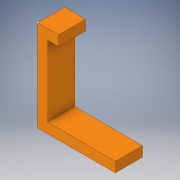
# Autodesk Inventor part: door stop supreme
Saved by Autodesk Inventor 2017 (Build 210142000, 142)
## iProperties
Created: 2018-09-26
Part Number: door stop supreme
Material: Generic
Document SubType Name: Modeling
Designer: Delta
Density: 1 g/cm^3
Appearance: Orange
Author: Delta
Autodesk Inventor part; units mm, degrees
ref_plane "YZ Plane" through (0, 0, 0) normal (1, 0, 0) x (0, 1, 0)
ref_plane "XZ Plane" through (0, 0, 0) normal (0, 1, 0) x (-1, 0, 0)
ref_plane "XY Plane" through (0, 0, 0) normal (0, 0, 1) x (1, 0, 0)
sketch "Sketch1" plane through (0, 0, 0) normal (0, 0, 1) x (1, 0, 0)
  line L0 (0, 0) -> (9.525, 0)
  line L1 (9.525, 0) -> (9.525, -95.25)
  line L2 (9.525, -95.25) -> (0, -95.25)
  line L3 (0, -95.25) -> (0, 0)
  dimension "d0" = 9.525
  dimension "d1" = 95.25
  constraints: 8 end point, 2 parallel, 1 horizontal, 1 perpendicular
  measures "d0" distance of L1.end L2.end
  measures "d1" distance of L0.end L1.end
extrude "Extrusion1" add sketch "Sketch1" along normal blind 25.4
sketch "Sketch2" plane through (9.525, -95.25, 0) normal (1, 0, 0) x (0, 0, -1)
  line L0 (-25.4, 95.25) -> (-25.4, 0) projected
  line L1 (0, 95.25) -> (-25.4, 95.25)
  line L2 (-25.4, 95.25) -> (-25.4, 85.725)
  line L3 (-25.4, 85.725) -> (0, 85.725)
  line L4 (0, 85.725) -> (0, 95.25)
  dimension "d4" = 9.525
  constraints: 8 end point, 2 parallel, 1 horizontal, 1 perpendicular, 1 point on line
  measures "d4" distance of L2.end L1.end
extrude "Extrusion2" add sketch "Sketch2" along normal blind 10.16
sketch "Sketch3" plane through (9.525, -95.25, 25.4) normal (1, 0, 0) x (0, 0, -1)
  line L0 (0, 0) -> (25.4, 0)
  line L1 (25.4, 0) -> (25.4, 9.525)
  line L2 (25.4, 9.525) -> (0, 9.525)
  line L3 (0, 9.525) -> (0, 0)
  point P0 (25.4, 95.25)
  dimension "d7" = 25.4
  dimension "d8" = 9.525
  constraints: 8 end point, 2 parallel, 1 horizontal, 1 perpendicular
  measures "d7" distance of L2.end L1.end
  measures "d8" distance of L1.end L0.end
extrude "Extrusion3" add sketch "Sketch3" along normal blind 63.5
sketch "Sketch4" plane through (0, 0, 25.4) normal (0, 0, 1) x (1, 0, 0)
  line L0 (73.025, -95.25) -> (73.025, -85.725) projected
  line L1 (0, 0) -> (0, -95.25) projected
  line L2 (73.025, -85.725) -> (0, -85.725)
  line L3 (0, -85.725) -> (0, -76.2)
  line L4 (0, -76.2) -> (73.025, -76.2)
  line L5 (73.025, -76.2) -> (73.025, -85.725)
  dimension "d11" = 9.525
  constraints: 8 end point, 2 parallel, 1 horizontal, 1 perpendicular, 1 point on line
  measures "d11" distance of L2.end L3.end
extrude "Extrusion4" add sketch "Sketch4" against normal blind 25.4
sketch "Sketch5" plane through (0, 0, 25.4) normal (0, 0, 1) x (1, 0, 0)
  line L0 (0, -95.25) -> (0, 0) projected
  line L1 (73.025, -95.25) -> (0, -95.25)
  line L2 (0, -95.25) -> (0, -85.725)
  line L3 (0, -85.725) -> (73.025, -85.725)
  line L4 (73.025, -85.725) -> (73.025, -95.25)
  dimension "d14" = 9.525
  constraints: 8 end point, 2 parallel, 1 horizontal, 1 perpendicular, 1 point on line
  measures "d14" distance of L1.end L2.end
extrude "Extrusion5" cut sketch "Sketch5" against normal blind 25.4
sketch "Sketch6" plane through (0, 0, 25.4) normal (0, 0, 1) x (1, 0, 0)
  point P0 (0, 0)
body "Solid1"
